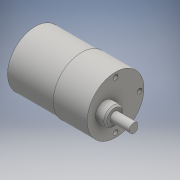
# Autodesk Inventor part: motor
Saved by Autodesk Inventor 2016 (Build 200138000, 138)
## iProperties
Created: 2015-09-14
Part Number: motor
Material: Generic
Document SubType Name: Modeling
Designer: Hulbert Office
Density: 1 g/cm^3
Appearance: Default
Author: Hulbert Office
Autodesk Inventor part; units mm, degrees
ref_plane "YZ Plane" through (0, 0, 0) normal (1, 0, 0) x (0, 1, 0)
ref_plane "XZ Plane" through (0, 0, 0) normal (0, 1, 0) x (-1, 0, 0)
ref_plane "XY Plane" through (0, 0, 0) normal (0, 0, 1) x (1, 0, 0)
sketch "Sketch1" plane through (0, 0, 0) normal (1, 0, 0) x (0, 1, 0)
  point P0 (0, 0)
sketch "Sketch2" plane through (0, 0, 0) normal (1, 0, 0) x (0, 1, 0)
  circle A0 centre (0, 0) radius 18.4
  dimension "d0" = 36.8
  constraints: 1 centre point, 1 coincident
  measures "d0" diameter of A0
extrude "Extrusion1" add sketch "Sketch2" along normal blind 22
sketch "Sketch3" plane through (22, 0, 0) normal (1, 0, 0) x (0, 0, -1)
  line L0 (0, 0) -> (0, -7)
  circle A0 centre (0, -7) radius 6
  dimension "d3" = 7
  dimension "d4" = 12
  constraints: 2 end point, 1 centre point, 1 coincident, 1 vertical
  measures "d3" distance of L0.start L0.end
  measures "d4" diameter of A0
extrude "Extrusion2" add sketch "Sketch3" along normal blind 6.4
chamfer "Chamfer1" distance 1 angle 45 1 edges at (28.4, -7, 6)
sketch "Sketch4" plane through (28.4, -7, 0) normal (1, 0, 0) x (0, 0, -1)
  circle A0 centre (0, 0) radius 5 projected
  circle A1 centre (0, 0) radius 3
  point P0 (0, 7)
  dimension "d10" = 6
  constraints: 1 centre point, 1 coincident
  measures "d10" diameter of A1
extrude "Extrusion3" add sketch "Sketch4" along normal blind 12.5 contours A1
sketch "Sketch5" plane through (40.9, -7, 0) normal (1, 0, 0) x (0, 0, -1)
  circle A0 centre (0, 0) radius 3 projected
  line L0 (0, -3) -> (0, 2.4)
  line L1 (0, 2.4) -> (1.8, 2.4)
  line L2 (-1.8, 2.4) -> (0, 2.4)
  point P0 (0, 7)
  dimension "d13" = 5.4
  constraints: 6 end point, 3 point on circle, 1 collinear, 1 perpendicular, 1 point on line, 1 vertical
  measures "d13" distance of L0.start L0.end
extrude "Extrusion4" cut sketch "Sketch5" against normal blind 12 contours L1 L2 A0
sketch "Sketch6" plane through (0, 0, 0) normal (-1, 0, 0) x (0, 0, 1)
  circle A0 centre (0, 0) radius 17.9
  dimension "d16" = 35.8
  constraints: 1 centre point, 1 coincident
  measures "d16" diameter of A0
extrude "Extrusion5" add sketch "Sketch6" along normal blind 30
sketch "Sketch9" plane through (22, 0, 0) normal (1, 0, 0) x (0, 0, -1)
  circle A0 centre (0, 0) radius 15.5
  circle A1 centre (0, 15.5) radius 1.5
  circle A2 centre (15.5, 0) radius 1.5
  circle A3 centre (-15.5, 0) radius 1.5
  dimension "d19" = 31
  dimension "d20" = 3
  dimension "d21" = 3
  dimension "d22" = 3
  constraints: 4 centre point, 3 point on circle, 1 coincident
  measures "d19" diameter of A0
  measures "d20" diameter of A1
  measures "d21" diameter of A2
  measures "d22" diameter of A3
extrude "Extrusion6" cut sketch "Sketch9" against normal blind 3 contours A0 A2 | A0 A2 | A1 A0 | A0 A1 | A3 A0 | A0 A3
body "Solid1"
